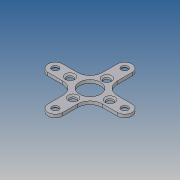
# Autodesk Inventor part: Motorkreuz_klein
Saved by Autodesk Inventor 2019.4 (Build 234330000, 330)
## iProperties
Part Number: Motorkreuz_klein
Material: GEDA Stahl
Document SubType Name: Modeling
Designer: Admin
Mass: 4.27907 g
Surface Area: 11.0239 cm^2
Volume: 0.54441 cm^3
Density: 7.86 g/cm^3
Appearance: GEDA Stahl A
Author: Admin
Gewicht: 0,004 kg
G_L: 0
G_H: 0
G_B: 0
InventorVersion: 2019.4
VAULT_Status: in Bearbeitung
Revision: -
Max. Breite: 0
Max. Höhe: 0
Max. Länge: 0
Max. Abmessungen: 0 x 0 x 0
Volumen: 544,41
Autodesk Inventor part; units mm, degrees
note: some values were not read from the file. Left out: dimensions or parameters whose unit could not be read.
ref_plane "YZ Plane" through (0, 0, 0) normal (1, 0, 0) x (0, 1, 0)
ref_plane "XZ Plane" through (0, 0, 0) normal (0, 1, 0) x (-1, 0, 0)
ref_plane "XY Plane" through (0, 0, 0) normal (0, 0, 1) x (1, 0, 0)
sketch "Skizze1" plane through (0, 0, 0) normal (0, 0, 1) x (1, 0, 0)
  line L0 (-20, -3.5) -> (20, -3.5)
  line L1 (20, -3.5) -> (20, 3.5)
  line L2 (20, 3.5) -> (-20, 3.5)
  line L3 (-20, 3.5) -> (-20, -3.5)
  line L4 (-20, -3.5) -> (20, 3.5) construction
  line L5 (20, -3.5) -> (-20, 3.5) construction
  line L6 (3.5, -20) -> (-3.5, -20)
  line L7 (-3.5, -20) -> (-3.5, 20)
  line L8 (-3.5, 20) -> (3.5, 20)
  line L9 (3.5, 20) -> (3.5, -20)
  line L10 (3.5, -20) -> (-3.5, 20) construction
  line L11 (-3.5, -20) -> (3.5, 20) construction
  point P0 (0, 0)
  dimension "d0" = 7
  dimension "d1" = 40
  constraints: 24 end point, 4 midpoint, 4 parallel, 4 perpendicular, 2 horizontal
  measures "d0" distance of L7.end L8.end
  measures "d1" distance of L8.end L6.start
extrude "Extrusion1" add sketch "Skizze1" along normal blind 1.5
fillet "Rundung1" radius 3.5 8 edges at (3.5, 20, 0.75) (-3.5, 20, 0.75) (20, 3.5, 0.75) (20, -3.5, 0.75) (3.5, -20, 0.75) (-3.5, -20, 0.75) (-20, -3.5, 0.75) (-20, 3.5, 0.75)
fillet "Rundung2" radius 6 4 edges at (3.5, 3.5, 0.75) (-3.5, 3.5, 0.75) (-3.5, -3.5, 0.75) (3.5, -3.5, 0.75)
sketch "Skizze2" plane through (0, 0, 1.5) normal (0, 0, 1) x (1, 0, 0)
  circle A0 centre (0, 0) radius 5
  circle A1 centre (16.5, 0) radius 1.6
  circle A2 centre (-16.5, 0) radius 1.6
  circle A3 centre (0, 16.5) radius 1.6
  circle A4 centre (0, -16.5) radius 1.6
  circle A5 centre (0, -8) radius 1.6
  circle A6 centre (0, 8) radius 1.6
  circle A7 centre (-9.5, 0) radius 1.6
  circle A8 centre (9.5, 0) radius 1.6
  line L0 (0, 16.5) -> (0, -16.5) construction
  line L1 (-16.5, 0) -> (16.5, 0) construction
  line L2 (9.5, 0) -> (-9.5, 0) construction
  line L3 (0, 8) -> (0, -8) construction
  dimension "d6" = 3.2
  dimension "d7" = 10
  dimension "d8" = 33
  dimension "d9" = 19
  dimension "d10" = 16
  constraints: 9 centre point, 8 end point, 7 equal radius, 5 midpoint, 4 vertical alignment, 3 horizontal alignment, 2 coincident, 2 collinear, 1 horizontal, 1 perpendicular, 1 vertical
  measures "d6" diameter of A1
  measures "d7" diameter of A0
  measures "d8" distance of L1.start L1.end
  measures "d9" distance of L2.end L2.start
  measures "d10" distance of L3.end L3.start
extrude "Extrusion2" cut sketch "Skizze2" against normal blind 1.5
chamfer "Fase1" distance 0.7 angle 45 4 edges at (-1.6, -8, 1.5) (-11.1, 0, 1.5) (-1.6, 8, 1.5) (7.9, 0, 1.5)
chamfer "Fase2" distance 0.7 angle 45 4 edges at (-1.6, 16.5, 0) (-18.1, 0, 0) (-1.6, -16.5, 0) (14.9, 0, 0)
equation "\"G_L\" = 0"
equation "\"G_H\" = 0"
equation "\"G_B\" = 0"
